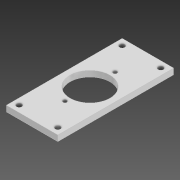
# Autodesk Inventor part: caster_holder
Saved by Autodesk Inventor 2020 (Build 240168000, 168)
## iProperties
Created: 2022-08-16
Part Number: caster_holder
Material: Generic
Document SubType Name: Modeling
Designer: Umair
Density: 1 g/cm^3
Appearance: Default
Author: Umair
Autodesk Inventor part; units mm, degrees
ref_plane "YZ Plane" through (0, 0, 0) normal (1, 0, 0) x (0, 1, 0)
ref_plane "XZ Plane" through (0, 0, 0) normal (0, 1, 0) x (-1, 0, 0)
ref_plane "XY Plane" through (0, 0, 0) normal (0, 0, 1) x (1, 0, 0)
sketch "Sketch1" plane through (0, 0, 0) normal (0, 1, 0) x (-1, 0, 0)
  line L0 (20, 45) -> (-20, 45)
  line L1 (-20, 45) -> (-20, -45)
  line L2 (-20, -45) -> (20, -45)
  line L3 (20, -45) -> (20, 45)
  line L4 (20, 45) -> (-20, -45) construction
  line L5 (-20, 45) -> (20, -45) construction
  circle A0 centre (0, 0) radius 15.5
  line L6 (0, 0) -> (0, -19.5)
  line L7 (0, -19.5) -> (0, 19.5)
  circle A1 centre (0, 19.5) radius 1.5
  circle A2 centre (0, -19.5) radius 1.5
  line L8 (15, 40) -> (-15, 40)
  line L9 (-15, 40) -> (-15, -40)
  line L10 (-15, -40) -> (15, -40)
  line L11 (15, -40) -> (15, 40)
  line L12 (15, 40) -> (-15, -40) construction
  line L13 (-15, 40) -> (15, -40) construction
  circle A3 centre (15, 40) radius 2
  circle A4 centre (15, -40) radius 2
  circle A5 centre (-15, -40) radius 2
  circle A6 centre (-15, 40) radius 2
  dimension "d0" = 40
  dimension "d1" = 90
  dimension "d2" = 31
  dimension "d3" = 19.5
  dimension "d4" = 39
  dimension "d5" = 3
  dimension "d6" = 3
  dimension "d9" = 30
  dimension "d10" = 80
  dimension "d11" = 4
  dimension "d12" = 4
  dimension "d13" = 4
  dimension "d14" = 4
  constraints: 28 end point, 7 centre point, 7 coincident, 4 midpoint, 4 parallel, 2 horizontal, 2 perpendicular, 1 point on line, 1 vertical
  measures "d0" distance of L2.end L1.end
  measures "d1" distance of L1.end L0.end
  measures "d2" diameter of A0
  measures "d3" distance of L6.start L6.end
  measures "d4" distance of L6.end L7.end
  measures "d5" diameter of A1
  measures "d6" diameter of A2
  measures "d9" distance of L10.end L9.end
  measures "d10" distance of L9.end L8.end
  measures "d11" diameter of A3
  measures "d12" diameter of A4
  measures "d13" diameter of A5
  measures "d14" diameter of A6
extrude "Extrusion1" add sketch "Sketch1" along normal blind 4.5 contours L3 L2 L1 L0 | A0 L9 A6 L8 A3 L11 | L11 A4 L10 A5 L9 A0
body "Solid1"
